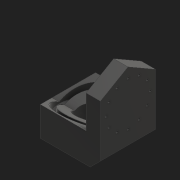
# Autodesk Inventor part: Arm L-Bracket
Saved by Autodesk Inventor 2017 (Build 210142000, 142)
## iProperties
Created: 2019-08-29
Part Number: Arm L-Bracket
Material: ABS Plastic
Document SubType Name: Modeling
Designer: Dell
Density: 1.06 g/cm^3
Appearance: Smooth - Black
Author: Dell
Autodesk Inventor part; units mm, degrees
ref_plane "YZ Plane" through (0, 0, 0) normal (1, 0, 0) x (0, 1, 0)
ref_plane "XZ Plane" through (0, 0, 0) normal (0, 1, 0) x (-1, 0, 0)
ref_plane "XY Plane" through (0, 0, 0) normal (0, 0, 1) x (1, 0, 0)
sketch "Sketch1" plane through (0, 0, 0) normal (0, 0, 1) x (1, 0, 0)
  line L0 (77.9423, 0) -> (38.9711, -67.5)
  line L1 (38.9711, -67.5) -> (-38.9711, -67.5)
  line L2 (-38.9711, -67.5) -> (-77.9423, 0)
  line L3 (-77.9423, 0) -> (-38.9711, 67.5)
  line L4 (-38.9711, 67.5) -> (38.9711, 67.5)
  line L5 (38.9711, 67.5) -> (77.9423, 0)
  line L6 (38.9711, 67.5) -> (47.9355, 67.5)
  line L7 (47.9355, 67.5) -> (102.9423, 67.5)
  line L8 (102.9423, 67.5) -> (102.9423, -67.5)
  line L9 (102.9423, -67.5) -> (38.9711, -67.5)
  circle A0 centre (0, 0) radius 22.5
  circle A1 centre (-54, 0) radius 2.5
  circle A2 centre (-46.7654, -27) radius 2.5
  circle A3 centre (-27, -46.7654) radius 2.5
  circle A4 centre (0, -54) radius 2.5
  circle A5 centre (27, -46.7654) radius 2.5
  circle A6 centre (46.7654, -27) radius 2.5
  circle A7 centre (54, 0) radius 2.5
  circle A8 centre (46.7654, 27) radius 2.5
  circle A9 centre (27, 46.7654) radius 2.5
  circle A10 centre (0, 54) radius 2.5
  circle A11 centre (-27, 46.7654) radius 2.5
  circle A12 centre (-46.7654, 27) radius 2.5
  dimension "d0" = 135
  dimension "d1" = 25
  dimension "d2" = 45
  dimension "d3" = 54
  dimension "d4" = 5
  dimension "d7" = 360
  constraints: 20 end point, 13 centre point, 2 coincident, 2 horizontal, 2 horizontal alignment, 1 perpendicular, 1 point on line, 38 other
  measures "d0" distance between parallel lines of L1 L4
  measures "d1" distance from line of L8 L0.start
  measures "d2" diameter of A0
  measures "d3" distance of point (0, 0) A1.centre
  measures "d4" diameter of A1
extrude "Extrusion1" add sketch "Sketch1" along normal blind 30
sketch "Sketch2" plane through (102.9423, -67.5, 0) normal (1, 0, 0) x (0, 0, -1)
  line L0 (-73.9711, 135) -> (-35, 67.5)
  line L1 (-35, 67.5) -> (-73.9711, 0)
  line L2 (-73.9711, 0) -> (-151.9134, 0)
  line L3 (-151.9134, 0) -> (-190.8846, 67.5)
  line L4 (-190.8846, 67.5) -> (-151.9134, 135)
  line L5 (-151.9134, 135) -> (-73.9711, 135)
  line L6 (0, 0) -> (0, 135) projected
  line L7 (0, 0) -> (-73.9711, 0)
  line L8 (0, 135) -> (-30, 135) projected
  line L9 (-73.9711, 135) -> (0, 135)
  line L10 (0, 135) -> (0, 0)
  circle A0 centre (-112.9423, 67.5) radius 22.5
  circle A1 centre (-166.9423, 67.5) radius 2.5
  circle A2 centre (-159.7077, 40.5) radius 2.5
  circle A3 centre (-139.9423, 20.7346) radius 2.5
  circle A4 centre (-112.9423, 13.5) radius 2.5
  circle A5 centre (-85.9423, 20.7346) radius 2.5
  circle A6 centre (-66.1769, 40.5) radius 2.5
  circle A7 centre (-58.9423, 67.5) radius 2.5
  circle A8 centre (-66.1769, 94.5) radius 2.5
  circle A9 centre (-85.9423, 114.2654) radius 2.5
  circle A10 centre (-112.9423, 121.5) radius 2.5
  circle A11 centre (-139.9423, 114.2654) radius 2.5
  circle A12 centre (-159.7077, 94.5) radius 2.5
  point P0 (0, 67.5)
  point P1 (-30, 0)
  dimension "d12" = 45
  dimension "d13" = 5
  dimension "d14" = 54
  dimension "d17" = 360
  dimension "d25" = 5
  constraints: 18 end point, 13 centre point, 3 horizontal alignment, 2 perpendicular, 1 coincident, 1 collinear, 1 horizontal, 38 other
  measures "d12" diameter of A0
  measures "d13" diameter of A1
  measures "d14" distance of point (-112.942, 67.5) A1.centre
  measures "d25" horizontal distance of L8.end L0.end
extrude "Extrusion2" add sketch "Sketch2" against normal blind 30 and the other way blind 5
sketch "Sketch3" plane through (72.9423, -67.5, 0) normal (-1, 0, 0) x (0, 0, 1)
  circle A0 centre (112.9423, 67.5) radius 22.5 projected
  line L0 (190.8846, 67.5) -> (151.9134, 0) projected
  line L1 (190.8846, 67.5) -> (151.9134, 0)
  line L2 (151.9134, 0) -> (73.9711, 0)
  line L3 (73.9711, 0) -> (35, 67.5)
  line L4 (35, 67.5) -> (73.9711, 135)
  line L5 (73.9711, 135) -> (151.9134, 135)
  line L6 (151.9134, 135) -> (190.8846, 67.5)
  line L7 (151.9134, 135) -> (30, 135) projected
  line L8 (73.9711, 135) -> (30, 135)
  line L9 (30, 0) -> (30, 135) projected
  line L10 (30, 135) -> (30, 0)
  line L11 (30, 0) -> (73.9711, 0)
  point P0 (0, 67.5)
  constraints: 18 end point, 2 collinear, 1 coincident, 1 perpendicular, 13 other
extrude "Extrusion3" add sketch "Sketch3" along normal blind 180 contours L11 L9 L7 L4 L3
sketch "Sketch4" plane through (0, 0, 0) normal (0, 0, -1) x (-1, 0, 0)
  line L0 (38.9711, -67.5) -> (-107.9423, -67.5) projected
  line L1 (77.9423, 0) -> (38.9711, -67.5) projected
  line L2 (38.9711, 67.5) -> (77.9423, 0) projected
  line L3 (38.9711, 67.5) -> (-107.9423, 67.5) projected
  line L4 (-107.9423, -67.5) -> (-107.9423, 67.5) construction
  circle A0 centre (0, 0) radius 22.5 projected
  circle A1 centre (46.7654, 27) radius 2.5 projected
  circle A2 centre (27, 46.7654) radius 2.5 projected
  circle A3 centre (0, 54) radius 2.5 projected
  circle A4 centre (-27, 46.7654) radius 2.5 projected
  circle A5 centre (-46.7654, 27) radius 2.5 projected
  circle A6 centre (-54, 0) radius 2.5 projected
  circle A7 centre (-46.7654, -27) radius 2.5 projected
  circle A8 centre (-27, -46.7654) radius 2.5 projected
  circle A9 centre (0, -54) radius 2.5 projected
  circle A10 centre (27, -46.7654) radius 2.5 projected
  circle A11 centre (46.7654, -27) radius 2.5 projected
  circle A12 centre (54, 0) radius 2.5 projected
  line L5 (38.9711, 67.5) -> (77.9423, 0) projected
  line L6 (77.9423, 0) -> (38.9711, -67.5) projected
  line L7 (38.9711, -67.5) -> (107.0577, -67.5) projected
  line L8 (107.0577, 67.5) -> (107.0577, -67.5) projected
  line L9 (38.9711, 67.5) -> (107.0577, 67.5) projected
extrude "Extrusion4" cut sketch "Sketch4" against normal through all
sketch "Sketch5" plane through (107.9423, -67.5, 0) normal (1, 0, 0) x (0, 0, -1)
  circle A0 centre (-112.9423, 67.5) radius 22.5
  point P0 (0, 67.5)
  constraints: 1 centre point
extrude "Extrusion5" add sketch "Sketch5" against normal blind 5
sketch "Sketch6" plane through (72.9423, -67.5, 0) normal (-1, 0, 0) x (0, 0, 1)
  circle A0 centre (112.9423, 67.5) radius 22.5 projected
  line L0 (92.6737, 77.2691) -> (48.2587, 90.4648)
  line L1 (90.4423, 67.5) -> (43.1177, 81.5602)
  line L2 (73.9711, 135) -> (35, 67.5) projected
  line L3 (73.9711, 135) -> (35, 67.5) projected
  circle A1 centre (66.1769, 94.5) radius 2.5 construction
  circle A2 centre (58.9423, 67.5) radius 2.5 construction
  circle A3 centre (66.1769, 94.5) radius 2.5 projected
  line L4 (66.1769, 94.5) -> (63.8542, 85.8314)
  line L5 (58.9423, 67.5) -> (61.265, 76.1686)
  line L6 (63.8542, 85.8314) -> (61.265, 76.1686) construction
  circle A4 centre (58.9423, 67.5) radius 2.5 projected
  line L7 (112.9423, 67.5) -> (58.9423, 67.5) construction
  line L8 (92.6737, 77.2691) -> (90.4423, 67.5)
  line L9 (48.2587, 90.4648) -> (43.1177, 81.5602)
  point P0 (0, 67.5)
  dimension "d30" = 10
  constraints: 16 end point, 5 point on line, 4 collinear, 2 point on circle, 1 horizontal, 1 parallel
  measures "d30" distance between parallel lines of L0 L1
extrude "Extrusion6" cut sketch "Sketch6" against normal blind 10 contours L8 A0 | A0 L1 L2 L0 picked at (91.27, 71.875)
sketch "Sketch7" plane through (-38.9711, 67.5, 73.9711) normal (0, -0.5, 0.8660254) x (1, 0, 0)
  ellipse E0 centre (38.9711, -77.9423) end of major axis (38.9711, -51.9615) minor radius 22.5 (61.4711, -77.9423) -> (16.4711, -77.9423) ccw projected
  line L0 (90.4711, -77.9423) -> (61.4711, -77.9423) projected
  ellipse E1 centre (92.9711, -77.9423) end of major axis (92.9711, -75.0555) minor radius 2.5 (95.4711, -77.9423) -> (90.4711, -77.9423) ccw projected
  line L1 (111.9134, -77.9423) -> (95.4711, -77.9423) projected
  line L2 (111.9134, -61.7069) -> (111.9134, -77.9423) projected
  line L3 (111.9134, -61.7069) -> (121.9134, -61.7069) projected
  line L4 (121.9134, -61.7069) -> (121.9134, -51.4248) projected
  line L5 (111.9134, -51.4248) -> (121.9134, -51.4248) projected
  line L6 (111.9134, 0) -> (111.9134, -51.4248) projected
  line L7 (111.9134, 0) -> (0, 0) projected
  line L8 (0, 0) -> (-38.9711, -77.9423) projected
  line L9 (-17.5289, -77.9423) -> (-38.9711, -77.9423) projected
  ellipse E2 centre (-15.0289, -77.9423) end of major axis (-15.0289, -75.0555) minor radius 2.5 (-12.5289, -77.9423) -> (-17.5289, -77.9423) ccw projected
  line L10 (16.4711, -77.9423) -> (-12.5289, -77.9423) projected
  ellipse E3 centre (85.7365, -46.7654) end of major axis (85.7365, -43.8786) minor radius 2.5 projected
  ellipse E4 centre (38.9711, -15.5885) end of major axis (38.9711, -12.7017) minor radius 2.5 projected
  ellipse E5 centre (-7.7942, -46.7654) end of major axis (-7.7942, -43.8786) minor radius 2.5 projected
  ellipse E6 centre (11.9711, -23.9423) end of major axis (11.9711, -21.0555) minor radius 2.5 projected
  ellipse E7 centre (65.9711, -23.9423) end of major axis (65.9711, -21.0555) minor radius 2.5 projected
  line L11 (111.9134, -61.7069) -> (61.4711, -77.9423)
  line L12 (92.9711, -77.9423) -> (90.782, -68.5083)
  line L13 (90.782, -68.5083) -> (88.5618, -58.9407) construction
  line L14 (88.5618, -58.9407) -> (85.7365, -46.7654)
  line L15 (111.9134, -51.4248) -> (59.8258, -68.1897)
  line L16 (59.8258, -68.1897) -> (61.4711, -77.9423)
  point P0 (38.9711, -95.4423)
  constraints: 12 end point, 3 point on line, 1 collinear, 1 parallel, 9 other
extrude "Extrusion7" cut sketch "Sketch7" against normal blind 10 contours E0 L15 L5 L4 L3 L11
ref_plane "Work Plane1" through (-38.9711, -67.5, 73.9711) normal (0, 0, -1) x (-1, 0, 0)
sketch "Sketch8" plane through (-38.9711, -67.5, 73.9711) normal (0, 0, -1) x (-1, 0, 0)
  circle A0 centre (-38.9711, 121.5) radius 2.5 projected
  circle A1 centre (-38.9711, 121.5) radius 6.5
  circle A2 centre (-38.9711, 67.5) radius 47.5
  circle A3 centre (-38.9711, 67.5) radius 22.5 projected
  circle A4 centre (-38.9711, 67.5) radius 60.5
  dimension "d36" = 13
  constraints: 3 centre point, 3 coincident, 2 tangent
  measures "d36" diameter of A1
extrude "Extrusion8" cut sketch "Sketch8" along normal blind 45 contours A0 | A1 | A4
chamfer "Chamfer1" distance 25 angle 45 1 edges at (107.9423, 0, 0)
sketch "Sketch9" plane through (72.9423, -67.5, 0) normal (-1, 0, 0) x (0, 0, 1)
  circle A0 centre (159.7077, 94.5) radius 2.5 construction
  circle A1 centre (139.9423, 114.2654) radius 2.5 construction
  circle A2 centre (112.9423, 121.5) radius 2.5 construction
  circle A3 centre (85.9423, 114.2654) radius 2.5 construction
  circle A4 centre (66.1769, 94.5) radius 2.5 construction
  circle A5 centre (58.9423, 67.5) radius 2.5 construction
  circle A6 centre (66.1769, 40.5) radius 2.5 construction
  circle A7 centre (85.9423, 20.7346) radius 2.5 construction
  circle A8 centre (112.9423, 13.5) radius 2.5 construction
  circle A9 centre (139.9423, 20.7346) radius 2.5 construction
  circle A10 centre (159.7077, 40.5) radius 2.5 construction
  circle A11 centre (166.9423, 67.5) radius 2.5 construction
  line L0 (90.4423, 67.5) -> (43.1177, 81.5602) construction
  line L1 (43.1177, 81.5602) -> (35, 67.5) construction
  line L2 (35, 67.5) -> (73.9711, 0) construction
  line L3 (73.9711, 0) -> (151.9134, 0) construction
  line L4 (151.9134, 0) -> (190.8846, 67.5) construction
  line L5 (190.8846, 67.5) -> (151.9134, 135) construction
  line L6 (151.9134, 135) -> (73.9711, 135) construction
  line L7 (73.9711, 135) -> (48.2587, 90.4648) construction
  line L8 (48.2587, 90.4648) -> (92.6737, 77.2691) construction
  arc A12 (90.4423, 67.5) -> (92.6737, 77.2691) centre (112.9423, 67.5) ccw construction
  line L9 (151.9134, 135) -> (190.8846, 67.5)
  line L10 (190.8846, 67.5) -> (151.9134, 0)
  line L11 (151.9134, 0) -> (73.9711, 0)
  line L12 (73.9711, 0) -> (35, 67.5)
  line L13 (35, 67.5) -> (73.9711, 135)
  line L14 (73.9711, 135) -> (151.9134, 135)
  line L15 (72.8164, 137) -> (32.6906, 67.5)
  line L16 (32.6906, 67.5) -> (72.8164, -2)
  line L17 (72.8164, -2) -> (153.0681, -2)
  line L18 (153.0681, -2) -> (193.194, 67.5)
  line L19 (193.194, 67.5) -> (153.0681, 137)
  line L20 (153.0681, 137) -> (72.8164, 137)
  point P0 (0, 67.5)
  dimension "d44" = 2
  constraints: 24 end point, 1 coincident, 18 other
  measures "d44" distance between parallel lines of L13 L15
extrude "Extrusion9" cut sketch "Sketch9" along normal through all contours L9 L10 L11 L12 L13 L14 | L20 L19 L18 L17 L16 L15
body "Solid1"
